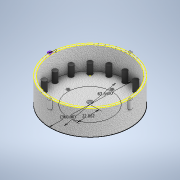
# Autodesk Inventor part: Joint
Saved by Autodesk Inventor 2021 (Build 250183000, 183)
## iProperties
Created: 2022-07-10
Part Number: Joint
Material: Ogólny
Document SubType Name: Modeling
Designer: MicnedSQ
Density: 1 g/cm^3
Appearance: Domyślna
Author: MicnedSQ
Autodesk Inventor part; units mm, degrees
ref_plane "YZ Plane" through (0, 0, 0) normal (1, 0, 0) x (0, 1, 0)
ref_plane "XZ Plane" through (0, 0, 0) normal (0, 1, 0) x (-1, 0, 0)
ref_plane "XY Plane" through (0, 0, 0) normal (0, 0, 1) x (1, 0, 0)
sketch "Szkic1" plane through (0, 0, 0) normal (0, 1, 0) x (-1, 0, 0)
  circle A0 centre (0, 0) radius 31.82
  circle A1 centre (0, 0) radius 40
  point P0 (0, 22.0617)
  point P1 (-22.0617, 0)
  point P2 (0, -22.0617)
  point P3 (22.0617, 0)
  dimension "d0" = 63.64
  dimension "d1" = 80
  dimension "d6" = 22.0617
  dimension "d9" = 360
  constraints: 4 coincident, 2 centre point, 5 other
  measures "d0" diameter of A0
  measures "d1" diameter of A1
  measures "d6" distance of point (0, 0) point (0, 22.062)
extrude "Wyciągnięcie proste1" add sketch "Szkic1" along normal blind 25 contours A0 | A1
shell "Skorupa1" thickness 2 removed faces 1 at (6.0893, 25, 16.5433)
hole "Otwór1" at (-22.0617, 0, 0) at (0, 0, 22.0617) at (22.0617, 0, 0) at (0, 0, -22.0617) direction (0, 1, 0) diameter 3 depth 6
hole "Otwór2" at (0, 0, 0) direction (0, 1, 0) diameter 5 depth 6
sketch "Szkic3" plane through (0, 2, 0) normal (0, 1, 0) x (1, 0, 0)
  circle A0 centre (0, 0) radius 2.5 projected
  circle A1 centre (0, 0) radius 35
  circle A2 centre (-35, 0) radius 2.45
  dimension "d35" = 70
  dimension "d36" = 4.9
  constraints: 1 centre point, 1 coincident, 1 horizontal alignment, 2 other
  measures "d36" diameter of A2
extrude "Wyciągnięcie proste3" add sketch "Szkic3" along normal blind 10 contours A2 A1 | A1 A2 picked at (-34.177, 0) picked at (-35.8041, 0.1006)
pattern_circular "Szyk kołowy1" count 16 over 360 about axis through (0, 0, 0) along (0, 1, 0) of "Wyciągnięcie proste3"
sketch "Szkic4" plane through (0, 25, 0) normal (0, 1, 0) x (1, 0, 0)
  circle A0 centre (0, 0) radius 40 projected
  circle A1 centre (-40, 0) radius 2
  circle A2 centre (0, 0) radius 38 projected
  circle A3 centre (-40, 0) radius 1
  dimension "d47" = 2
  constraints: 2 centre point, 1 coincident, 1 horizontal alignment, 1 tangent, 1 other
  measures "d47" diameter of A3
extrude "Wyciągnięcie proste4" add sketch "Szkic4" against normal blind 10 contours A1 A0 A3 | A0 A3 A1 | A3 A0 | A0 A3
extrude "Wyciągnięcie proste5" cut sketch "Szkic4" against normal blind 6 contours A3 A0 | A0 A3
fillet "Zaokrąglenie1" radius 2 1 edges at (-42, 15, 0)
pattern_circular "Szyk kołowy3" count 4 over 360 about axis through (0, 0, 0) along (0, 1, 0) of "Wyciągnięcie proste4", "Wyciągnięcie proste5", "Zaokrąglenie1"
